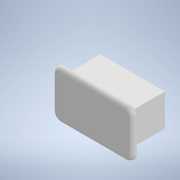
# Autodesk Inventor part: button
Saved by Autodesk Inventor 2022 (Build 260153000, 153)
## iProperties
Created: 2020-11-05
Part Number: button
Material: Generic
Document SubType Name: Modeling
Designer: simen
Density: 1 g/cm^3
Appearance: Default
Author: simen
## iProperties of the stored document button_3DPrint.ipt
Created: 2021-12-01
Part Number: button_3DPrint
Material: Generic
Document SubType Name: Modeling
Designer: simen
Density: 1 g/cm^3
Appearance: Default
Author: simen
Autodesk Inventor part; units mm, degrees
ref_plane "YZ Plane" through (0, 0, 0) normal (1, 0, 0) x (0, 1, 0)
ref_plane "XZ Plane" through (0, 0, 0) normal (0, 1, 0) x (-1, 0, 0)
ref_plane "XY Plane" through (0, 0, 0) normal (0, 0, 1) x (1, 0, 0)
sketch "Sketch1" plane through (0, 0, 0) normal (0, 0, 1) x (1, 0, 0)
  circle A0 centre (10.6405, 2.5912) radius 4
  line L0 (15.6405, 6.5912) -> (5.6405, 6.5912)
  line L1 (4.6405, 5.5912) -> (4.6405, -0.4088)
  line L2 (5.6405, -1.4088) -> (15.6405, -1.4088)
  line L3 (16.6405, -0.4088) -> (16.6405, 5.5912)
  line L4 (16.6405, 6.5912) -> (4.6405, -1.4088) construction
  line L5 (4.6405, 6.5912) -> (16.6405, -1.4088) construction
  arc A1 (5.6405, 6.5912) -> (4.6405, 5.5912) centre (5.6405, 5.5912) ccw
  arc A2 (4.6405, -0.4088) -> (5.6405, -1.4088) centre (5.6405, -0.4088) ccw
  arc A3 (15.6405, -1.4088) -> (16.6405, -0.4088) centre (15.6405, -0.4088) ccw
  arc A4 (16.6405, 5.5912) -> (15.6405, 6.5912) centre (15.6405, 5.5912) ccw
  point P0 (0, 0)
  point P1 (10.6405, 6.5912)
  point P2 (10.6405, -1.4088)
  dimension "d6" = 8
  dimension "d13" = 8
  dimension "d14" = 12
  dimension "d15" = 1
  constraints: 12 end point, 8 point on circle, 8 point on line, 8 tangent, 5 centre point, 3 equal radius, 2 midpoint, 2 parallel, 1 horizontal, 1 perpendicular
  measures "d6" diameter of A0
  measures "d13" distance of L4.end L5.start
  measures "d14" distance of L4.start L5.start
  measures "d15" radius of A1
extrude "Extrusion1" add sketch "Sketch1" along normal blind 1
sketch "Sketch2" plane through (10.6405, 2.5912, 0) normal (0, 0, -1) x (-1, 0, 0)
  circle A0 centre (0, 0) radius 3
  line L0 (5, -4) -> (-5, -4) projected
  arc A1 (-6, -3) -> (-5, -4) centre (-5, -3) ccw projected
  line L1 (-6, -3) -> (-6, 3) projected
  arc A2 (-5, 4) -> (-6, 3) centre (-5, 3) ccw projected
  line L2 (-5, 4) -> (5, 4) projected
  arc A3 (6, 3) -> (5, 4) centre (5, 3) ccw projected
  line L3 (6, 3) -> (6, -3) projected
  arc A4 (5, -4) -> (6, -3) centre (5, -3) ccw projected
  line L4 (-4, -3) -> (4, -3)
  line L5 (5, -2) -> (5, 2)
  line L6 (4, 3) -> (-4, 3)
  line L7 (-5, 2) -> (-5, -2)
  arc A5 (5, 2) -> (4, 3) centre (4, 2) ccw
  arc A6 (4, -3) -> (5, -2) centre (4, -2) ccw
  arc A7 (-5, -2) -> (-4, -3) centre (-4, -2) ccw
  arc A8 (-4, 3) -> (-5, 2) centre (-4, 2) ccw
  point P0 (10.6405, -2.5912)
  point P1 (0, 3)
  point P2 (0, -3)
  dimension "d16" = 1
  dimension "d17" = 1
  constraints: 8 end point, 8 point on circle, 8 tangent, 5 centre point, 3 equal radius, 3 other
  measures "d16" distance between parallel lines of L0 L4
  measures "d17" radius of A5
extrude "Extrusion2" add sketch "Sketch2" along normal blind 1.3 and the other way blind 3.5 contours A0 | A0 L6 A5 L5 A6 L4 | A0 L4 A7 L7 A8 L6
fillet "Fillet3" radius 0.5 10 edges at (15.3476, -0.1159, 3.5) (15.6405, 2.5912, 3.5) (15.3476, 5.2983, 3.5) (12.6405, 5.5912, 3.5) (8.6405, 5.5912, 3.5) (5.9334, 5.2983, 3.5) (5.6405, 2.5912, 3.5) (5.9334, -0.1159, 3.5) (8.6405, -0.4088, 3.5) (12.6405, -0.4088, 3.5)
sketch "Sketch4" plane through (0, 0, 0) normal (0, 0, -1) x (-1, 0, 0)
  point P0 (0, 0)
sketch "Sketch6" plane through (0, 0, 0) normal (0, 0, -1) x (-1, 0, 0)
  arc A0 (-15.6405, 0.5912) -> (-14.6405, -0.4088) centre (-14.6405, 0.5912) ccw projected
  line L0 (-15.6405, 0.5912) -> (-15.6405, 4.5912) projected
  arc A1 (-14.6405, 5.5912) -> (-15.6405, 4.5912) centre (-14.6405, 4.5912) ccw projected
  line L1 (-14.6405, 5.5912) -> (-6.6405, 5.5912) projected
  arc A2 (-5.6405, 4.5912) -> (-6.6405, 5.5912) centre (-6.6405, 4.5912) ccw projected
  line L2 (-5.6405, 4.5912) -> (-5.6405, 0.5912) projected
  arc A3 (-6.6405, -0.4088) -> (-5.6405, 0.5912) centre (-6.6405, 0.5912) ccw projected
  line L3 (-6.6405, -0.4088) -> (-14.6405, -0.4088) projected
  line L4 (-5.6405, -1.4088) -> (-15.6405, -1.4088) projected
  arc A4 (-5.6405, -1.4088) -> (-4.6405, -0.4088) centre (-5.6405, -0.4088) ccw projected
  line L5 (-4.6405, 5.5912) -> (-4.6405, -0.4088) projected
  arc A5 (-4.6405, 5.5912) -> (-5.6405, 6.5912) centre (-5.6405, 5.5912) ccw projected
  line L6 (-15.6405, 6.5912) -> (-5.6405, 6.5912) projected
  arc A6 (-15.6405, 6.5912) -> (-16.6405, 5.5912) centre (-15.6405, 5.5912) ccw projected
  line L7 (-16.6405, -0.4088) -> (-16.6405, 5.5912) projected
  arc A7 (-16.6405, -0.4088) -> (-15.6405, -1.4088) centre (-15.6405, -0.4088) ccw projected
  point P0 (0, 0)
extrude "Extrusion5" add sketch "Sketch6" along normal up to surface (1.3 mm away)
sketch "Sketch7" plane through (10.6405, 2.5912, -1.3) normal (0, 0, -1) x (-1, 0, 0)
  arc A0 (6, 3) -> (5, 4) centre (5, 3) ccw projected
  line L0 (-5, 4) -> (5, 4) projected
  arc A1 (-5, 4) -> (-6, 3) centre (-5, 3) ccw projected
  line L1 (-6, -3) -> (-6, 3) projected
  arc A2 (-6, -3) -> (-5, -4) centre (-5, -3) ccw projected
  line L2 (5, -4) -> (-5, -4) projected
  arc A3 (5, -4) -> (6, -3) centre (5, -3) ccw projected
  line L3 (6, 3) -> (6, -3) projected
  line L4 (4, -2) -> (-4, -2)
  line L5 (-4, -2) -> (-4, 2)
  line L6 (-4, 2) -> (4, 2)
  line L7 (4, 2) -> (4, -2)
  point P0 (10.6405, -2.5912)
  dimension "d28" = 2
  constraints: 8 end point, 3 other
  measures "d28" distance between parallel lines of L3 L7
extrude "Extrusion6" cut sketch "Sketch7" against normal blind 1.5
chamfer "Chamfer2" distance 1.5 angle 45 4 edges at (10.6405, 0.5912, 0.2) (6.6405, 2.5912, 0.2) (10.6405, 4.5912, 0.2) (14.6405, 2.5912, 0.2)
body "Solid1"
